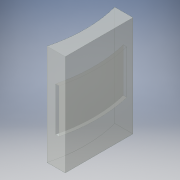
# Autodesk Inventor part: Cover
Saved by Autodesk Inventor 2016 (Build 200138000, 138)
## iProperties
Created: 2016-05-27
Part Number: Cover
Material: Glass
Document SubType Name: Modeling
Designer: xdlea
Density: 2.18 g/cm^3
Appearance: Clear
Author: xdlea
Autodesk Inventor part; units mm, degrees
ref_plane "YZ Plane" through (0, 0, 0) normal (1, 0, 0) x (0, 1, 0)
ref_plane "XZ Plane" through (0, 0, 0) normal (0, 1, 0) x (-1, 0, 0)
ref_plane "XY Plane" through (0, 0, 0) normal (0, 0, 1) x (1, 0, 0)
sketch "Sketch1" plane through (0, 0, 0) normal (0, 1, 0) x (-1, 0, 0)
  line L0 (0, 20.193) -> (0, -20.193)
  line L1 (0, -20.193) -> (3.6912, -20.193)
  line L2 (0, 20.193) -> (3.6912, 20.193)
  arc A0 (10.8286, 20.193) -> (10.8286, -20.193) centre (86.8455, 0) ccw
  arc A1 (5.7486, 20.193) -> (5.7486, -20.193) centre (86.8455, 0) ccw
  arc A2 (3.6912, 20.193) -> (3.6912, -20.193) centre (86.8455, 0) ccw
  line L3 (5.7486, 20.193) -> (10.8286, 20.193)
  line L4 (3.6912, 20.193) -> (5.7486, 20.193)
  line L5 (3.6912, -20.193) -> (5.7486, -20.193)
  line L6 (5.7486, -20.193) -> (10.8286, -20.193)
  point P0 (0, 0)
  point P1 (8.1923, 0)
  point P2 (0, 0)
  dimension "d0" = 2.0574
  dimension "d1" = 5.08
  dimension "d2" = 8.1923
  dimension "d3" = 40.386
  dimension "d4" = 10.8286
  constraints: 14 end point, 7 point on circle, 3 centre point, 3 coincident, 3 horizontal, 3 perpendicular, 1 horizontal alignment, 1 midpoint, 1 point on line, 1 vertical
  measures "d0" distance of L1.end L5.end
  measures "d1" distance of L5.end L6.end
  measures "d2" distance from line of L0 point (8.192, 0)
  measures "d3" distance of L0.start L0.end
  measures "d4" distance from line of L6.end L0
extrude "Extrusion1" add sketch "Sketch1" along normal mid plane 60.1218
extrude "Extrusion2" cut sketch "Sketch1" along normal mid plane 26.162 contours L4 A1 L5 A2
equation "\"d2\" = LowerArch"
equation "\"d4\" = Height"
equation "\"Height\" = 10.828576"
equation "\"LowerArch\" = 8.192275"
body "Solid1"
